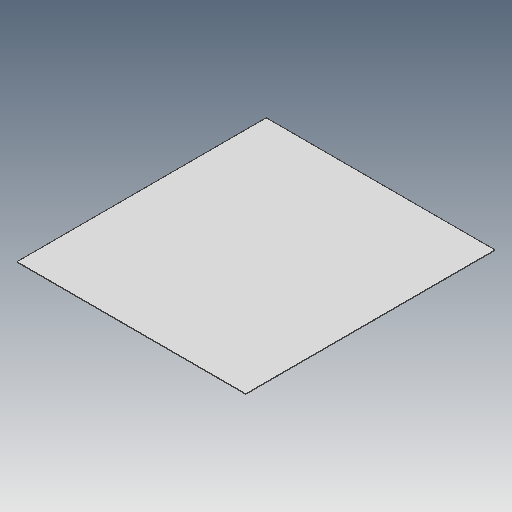
# Autodesk Inventor part: side_panel_actual
Saved by Autodesk Inventor 2027 (Build 310192060, 192F)
## iProperties
Created: 2026-07-27
Part Number: side_panel_actual
Material: Generic
Document SubType Name: Sheet Metal
Designer: prest
Density: 1 g/cm^3
Sheet Metal Rule: Default_mm
Appearance: Default
Author: prest
Autodesk Inventor part; units mm, degrees
ref_plane "YZ Plane" through (0, 0, 0) normal (1, 0, 0) x (0, 1, 0)
ref_plane "XZ Plane" through (0, 0, 0) normal (0, 1, 0) x (-1, 0, 0)
ref_plane "XY Plane" through (0, 0, 0) normal (0, 0, 1) x (1, 0, 0)
sketch "Sketch1" plane through (0, 0, 0) normal (0, 1, 0) x (-1, 0, 0)
  line L0 (111.8, 121.8) -> (-111.8, 121.8)
  line L1 (-111.8, 121.8) -> (-111.8, -121.8)
  line L2 (-111.8, -121.8) -> (111.8, -121.8)
  line L3 (111.8, -121.8) -> (111.8, 121.8)
  point P0 (0, 0)
  point P1 (111.8, 0)
  point P2 (0, -121.8)
  dimension "d0" = 223.6
  dimension "d1" = 243.6
  measures "d0" distance of L0.start L0.end
  measures "d1" distance of L0.end L1.end
extrude "Plate1" add sketch "Sketch1" along normal blind 0.5
equation "\"d2\" = Thickness"
equation "\"BendRadius\" = Thickness"
equation "\"BendReliefWidth\" = Thickness"
equation "\"BendReliefDepth\" = 0.5 * Thickness"
equation "\"CornerReliefSize\" = 4 * Thickness"
equation "\"MinimumRemnant\" = 2 * Thickness"
equation "\"TransitionRadius\" = BendRadius"
equation "\"JacobiRadiusSize\" = BendRadius"
equation "\"GapSize\" = Thickness"
equation "\"Thickness\" = 0.5"
body "Solid1"
